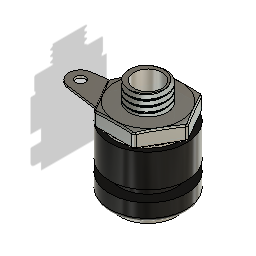
4mm Black Banana Female Socket Jack Mount Connectors (Autodesk Fusion 360 design; units mm, degrees)
Autodesk Fusion 360 part; units mm, degrees
note: some values were not read from the file. Set by a fixed rule: which sketch regions a step uses.
sketch "Sketch1" plane through (0, 0, 0) normal (0, 0, 1) x (1, 0, 0)
  circle A0 centre (0, 0) radius 4
  circle A1 centre (0, 0) radius 2
  circle A2 centre (0, 0) radius 2.7
  circle A3 centre (0, 0) radius 2.8
  dimension "d1" = 8
  dimension "d2" = 4
  dimension "d3" = 5.4
  dimension "d6" = 5.6
  constraint coincident A0.centre A1.centre
  constraint concentric A0 A2
  measures "d1" diameter of A0
  measures "d2" diameter of A1
  measures "d3" diameter of A2
  measures "d6" diameter of A3
extrude "Extrude1" add sketch "Sketch1" along normal blind 1.1 contours A0 | A2 | A3 picked at (3.585108, -0.198723) picked at (2.449168, -0.2335) picked at (-2.592788, -0.945343) makes body 1
extrude "Extrude2" add sketch "Sketch1" along normal blind 15 contours A2 | A3 picked at (2.449168, -0.2335) picked at (-2.592788, -0.945343) bodies 1
chamfer "Chamfer1" distance 0.75 angle 45 1 edges at (-1.864655, 0.723231, 0) on bodies 1
thread "Thread1" "ANSI Unified Screw Threads 0.216(#12) 12-32 UNEF 3A" major diameter 5.4102 minor diameter 4.54152 pitch 0.79375 angle 60 modelled right hand crest width 0.125578 on face at (2.786086, 0.27879, 5.733333) crest through (2.7051, 0, 0.901563) on bodies 1
sketch "Sketch3" plane through (0, 0, 1.1) normal (0, 0, 1) x (1, 0, 0)
  arc A0 (1.289831, 2.377794) -> (-1.289831, 2.377794) centre (0, 0) ccw
  spline S0 degree 3 poles (1.289831, 2.377794) (1.45532, 2.269904) (1.60845, 2.144156) (1.881451, 1.863469) (2.001034, 1.709933) (2.276488, 1.260579) (2.394339, 0.945861) (2.499052, 0.299459) (2.489009, -0.025287) (2.345553, -0.641531) (2.217586, -0.927994) (1.863779, -1.425664) (1.644761, -1.634456) (1.391422, -1.794518) knots -0.49614536 -0.49614536 -0.49614536 -0.49614536 -0.43707144 -0.43707144 -0.37904408 -0.37904408 -0.27942365 -0.27942365 -0.18304181 -0.18304181 -0.08990008 -0.08990008 0 0 0 0
  arc A1 (-1.391422, -1.794518) -> (1.391422, -1.794518) centre (0, 0) ccw
  spline S1 degree 3 poles (-1.391422, -1.794518) (-1.533964, -1.704459) (-1.665988, -1.598735) (-1.907097, -1.357971) (-2.014904, -1.223126) (-2.274325, -0.813896) (-2.38751, -0.51945) (-2.498549, 0.106872) (-2.491225, 0.433391) (-2.351413, 1.076556) (-2.216212, 1.386071) (-1.830095, 1.946169) (-1.579499, 2.188947) (-1.289831, 2.377794) knots -0.49798717 -0.49798717 -0.49798717 -0.49798717 -0.44724423 -0.44724423 -0.39545761 -0.39545761 -0.30146729 -0.30146729 -0.20422667 -0.20422667 -0.1037371 -0.1037371 0 0 0 0
  circle A2 centre (0, 0) radius 4
  circle A3 centre (0, 0) radius 5.5
  circle A4 centre (0, 0) radius 3.05
  circle A5 centre (0, 0) radius 4
  dimension "d11" = 11
  dimension "d12" = 6.1
  dimension "d13" = 8
  constraint coincident A0.centre A1.centre
  constraint concentric A4 A5
  measures "d11" diameter of A3
  measures "d12" diameter of A4
  measures "d13" diameter of A5
extrude "Extrude3" add sketch "Sketch3" along normal blind 7 separate body contours A2 A5 picked at (3.657086, -0.350249) makes body 2
extrude "Extrude4" add sketch "Sketch3" along normal blind 2.55 contours A3 picked at (4.964631, -0.471967) bodies 2
fillet "Fillet1" radius 0.6 1 edges at (-5.1278, -1.988885, 1.1) on bodies 2
sketch "Sketch4" plane through (0, 0, 3.65) normal (0, 0, 1) x (1, 0, 0)
  circle A0 centre (0, 0) radius 4
  circle A1 centre (0, 0) radius 5.5
  circle A2 centre (0, 0) radius 4.025
  circle A3 centre (0, 0) radius 5.5
  dimension "d20" = 8.05
  constraint coincident A0.centre A1.centre
  constraint concentric A2 A3
  measures "d20" diameter of A2
extrude "Extrude5" add sketch "Sketch4" along normal blind 4.7 separate body contours A1 A3 picked at (4.972871, -0.473209) makes body 3
sketch "Sketch5" plane through (0, 0, 8.35) normal (0, 0, 1) x (1, 0, 0)
  circle A0 centre (0, 0) radius 4.025
  circle A1 centre (0, 0) radius 5.5
  circle A2 centre (0, 0) radius 3.225
  circle A3 centre (0, 0) radius 4.8
  line L0 (2.5, -6.039835) -> (-2.5, -6.039835) construction
  line L1 (2.5, -6.039835) -> (-2.5, 6.039835) construction
  line L2 (-2.5, -6.039835) -> (2.5, 6.039835) construction
  line L3 (2.5, -4.09756) -> (2.5, -6.039835) construction
  line L4 (-2.5, -6.039835) -> (-2.5, -4.09756) construction
  line L5 (0, 0) -> (0, 4.8) construction
  line L6 (0, 4.8) -> (0, -11.4) construction
  line L7 (0, -11.4) -> (0, -9.7)
  circle A4 centre (0, -9.7) radius 1.7
  line L8 (2.5, -4.09756) -> (1.683617, -9.935441)
  line L9 (-2.5, -4.09756) -> (-1.683617, -9.935441)
  circle A5 centre (0, -9.7) radius 0.7
  dimension "d23" = 6.45
  dimension "d24" = 9.6
  dimension "d25" = 5
  dimension "d26" = 16.2
  dimension "d27" = 1.7
  dimension "d28" = 1.4
  constraint coincident A0.centre A1.centre
  constraint concentric A2 A3
  constraint horizontal L0
  constraint perpendicular L0 L4
  constraint coincident L1 A0.centre
  constraint coincident L2 A0.centre
  constraint coincident A3 L5.end
  constraint vertical L5
  constraint perpendicular L0 L6
  constraint parallel L6 L7
  constraint coincident L7.end A4.centre
  constraint coincident L6.end A4
  constraint tangent A4 L8
  constraint tangent A4 L9
  constraint concentric A4 A5
  measures "d23" diameter of A2
  measures "d24" diameter of A3
  measures "d26" distance of L5.end L6.end
  measures "d27" distance of L6.end L7.end
  measures "d28" diameter of A5
extrude "Extrude6" add sketch "Sketch5" along normal blind 0.3 separate body contours A0 | A1 A3 L8 L9 | A1 A4 L8 L9 | A3 | A4 picked at (3.731341, -0.360185) picked at (1.971039, -4.872073) picked at (0.400922, -6.327743) picked at (-2.696383, -3.642095) picked at (-1.360053, -9.795586) makes body 4
fillet "Fillet2" radius 0.2 2 edges at (2.5, -4.09756, 8.5) (-2.5, -4.09756, 8.5) on bodies 4
sketch "Sketch6" plane through (0, 0, 8.65) normal (0, 0, 1) x (1, 0, 0)
  circle A0 centre (0, 0) radius 3.225
  circle A1 centre (0, -9.7) radius 0.7
  arc A2 (2.577722, -4.049117) -> (-2.577722, -4.049117) centre (0, 0) ccw
  arc A3 (-2.487055, -4.190131) -> (-2.577722, -4.049117) centre (-2.685127, -4.21783) ccw
  line L0 (-2.487055, -4.190131) -> (-1.683617, -9.935441)
  arc A4 (-1.683617, -9.935441) -> (1.683617, -9.935441) centre (0, -9.7) ccw
  line L1 (1.683617, -9.935441) -> (2.487055, -4.190131)
  arc A5 (2.577722, -4.049117) -> (2.487055, -4.190131) centre (2.685127, -4.21783) ccw
  line L2 (4.95, 2.857884) -> (0, 5.715768)
  line L3 (0, 5.715768) -> (-4.95, 2.857884)
  line L4 (-4.95, 2.857884) -> (-4.95, -2.857884)
  line L5 (-4.95, -2.857884) -> (0, -5.715768)
  line L6 (0, -5.715768) -> (4.95, -2.857884)
  line L7 (4.95, -2.857884) -> (4.95, 2.857884)
  circle A6 centre (0, 0) radius 2.725
  dimension "d33" = 4.95
  dimension "d34" = 5.45
  constraint coincident A0.centre A2.centre
  measures "d33" distance of A0.centre L7
  measures "d34" diameter of A6
extrude "Extrude7" add sketch "Sketch6" along normal blind 2.12 separate body contours A0 | A2 A3 L0 L1 A5 L5 L6 | A2 A3 L0 L1 A5 L2 L3 L4 L5 L6 L7 picked at (3.036181, -0.2956) picked at (-1.063678, -4.382552) picked at (0, 5.096601) makes body 5
fillet "Fillet3" radius 0.5 6 edges at (4.95, 2.857884, 9.71) (0, 5.715768, 9.71) (-4.95, 2.857884, 9.71) (-4.95, -2.857884, 9.71) (0, -5.715768, 9.71) (4.95, -2.857884, 9.71) on bodies 5
fillet "Fillet4" radius 0.2 12 edges at (2.475, 4.286826, 8.65) (0, 5.638417, 8.65) (-2.475, 4.286826, 8.65) (-4.883013, 2.819209, 8.65) (-4.95, 0, 8.65) (-4.883013, -2.819209, 8.65) (-2.475, -4.286826, 8.65) (0, -5.638417, 8.65) (2.475, -4.286826, 8.65) (4.883013, -2.819209, 8.65) (4.95, 0, 8.65) (4.883013, 2.819209, 8.65) on bodies 5
sketch "Sketch7" plane through (0, 0, 0) normal (0, 1, 0) x (1, 0, 0)
  line L0 (0, -10.77) -> (0.1, -10.77)
  line L1 (2.725, -10.77) -> (-2.725, -10.77)
  line L2 (2.725, -10.77) -> (4.75, -10.77)
  line L3 (0, -10.77) -> (5.638417, -10.77)
  line L4 (5.638417, -10.77) -> (5.638417, -10.62)
  arc A0 (4.75, -10.77) -> (5.638417, -10.62) centre (4.75, -8.064048) ccw
  dimension "d41" = 2.025
  dimension "d43" = 5.638417
  dimension "d44" = 0.15
  constraint coincident L1.start L2.start
  constraint parallel L1 L3
  constraint perpendicular L3 L4
  constraint tangent L2 A0
  measures "d41" distance of L1.start L2.end
sketch "Sketch8" plane through (0, 0, 10.77) normal (0, 0, 1) x (1, 0, 0)
  arc A0 (4.7, -3.002221) -> (4.95, -2.569209) centre (4.45, -2.569209) ccw
  line L0 (4.95, -2.569209) -> (4.95, 2.569209)
  arc A1 (4.95, 2.569209) -> (4.7, 3.002221) centre (4.45, 2.569209) ccw
  line L1 (4.7, 3.002221) -> (0.25, 5.57143)
  arc A2 (0.25, 5.57143) -> (-0.25, 5.57143) centre (0, 5.138417) ccw
  line L2 (-0.25, 5.57143) -> (-4.7, 3.002221)
  arc A3 (-4.7, 3.002221) -> (-4.95, 2.569209) centre (-4.45, 2.569209) ccw
  line L3 (-4.95, 2.569209) -> (-4.95, -2.569209)
  arc A4 (-4.95, -2.569209) -> (-4.7, -3.002221) centre (-4.45, -2.569209) ccw
  line L4 (-4.7, -3.002221) -> (-0.25, -5.57143)
  arc A5 (-0.25, -5.57143) -> (0.25, -5.57143) centre (0, -5.138417) ccw
  line L5 (0.25, -5.57143) -> (4.7, -3.002221)
  circle A6 centre (0, 0) radius 2.725
revolve "Revolve1" cut sketch "Sketch7" angle 360 about axis through (0, 0, 8.65) along (0, 0, -1) bodies 5
fillet "Fillet5" radius 0.2 18 edges at (-4.933066, -2.698236, 10.625386) (-4.95, 0, 10.762599) (-4.933077, 2.698197, 10.625392) (-4.803274, 2.923043, 10.625386) (-2.475, 4.286826, 10.762599) (-0.129831, 5.621269, 10.625392) (0.129792, 5.621279, 10.625386) (2.475, 4.286826, 10.762599) (4.803246, 2.923072, 10.625392) (4.933066, 2.698236, 10.625386) (4.95, 0, 10.762599) (4.933077, -2.698197, 10.625392) (4.803274, -2.923043, 10.625386) (2.475, -4.286826, 10.762599) (0.129831, -5.621269, 10.625392) (-0.129792, -5.621279, 10.625386) (-2.475, -4.286826, 10.762599) (-4.803246, -2.923072, 10.625392) on bodies 5
move_body "Move1" bodies 4 5 3 to x (1, 0, 0) y (0, 1, 0) z (0, 0, 1) at (0, 0, 1.6)
equation "d27 = ( 3.4 / 2 ) * 1 mm"
equation "d33 = ( 9.9 / 2 ) * 1 mm"
equation "d43 = 11.27683479 mm / 2"
